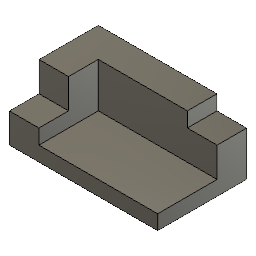
_Practice2.af6316e0-147c-47ba-990e-6d72fd886336 (Autodesk Fusion 360 design; units mm, degrees)
Autodesk Fusion 360 part; units mm, degrees
sketch "Sketch1" plane through (0, 0, 0) normal (0, 0, 1) x (1, 0, 0)
  line L0 (4, 0) -> (0, 0)
  line L1 (0, 0) -> (0, 2.25)
  line L2 (0, 2.25) -> (1.5, 2.25)
  line L3 (1.5, 2.25) -> (1.5, 1.5)
  line L4 (1.5, 1.5) -> (2.75, 1.5)
  line L5 (2.75, 1.5) -> (2.75, 0.75)
  line L6 (2.75, 0.75) -> (4, 0.75)
  line L7 (4, 0.75) -> (4, 0)
  dimension "d1" = 4
  dimension "d4" = 2.25
  dimension "d5" = 1.25
  dimension "d6" = 1.5
  dimension "d7" = 0.75
  dimension "d8" = 0.75
  dimension "d10" = 1.25
  measures "d1" distance of L0.end
  measures "d4" distance of L0.end
sketch "Sketch2" plane through (0, 2.25, 0) normal (0, 1, 0) x (-1, 0, 0)
  line L0 (-1.5, 0) -> (0, 0)
  line L1 (0, 0) -> (0, 1.25)
  line L2 (0, 1.25) -> (-1.5, 1.25)
  line L3 (-1.5, 1.25) -> (-1.5, 0)
  line L4 (-1.5, 0.2963) -> (-0.6318, 0.2963)
  line L5 (-0.6318, 0.2963) -> (-0.6318, 0.976)
  line L6 (-0.6318, 0.976) -> (-3.3284, 0.976)
  line L7 (-3.3284, 0.976) -> (-3.3284, 0.2963)
  line L8 (-3.3284, 0.2963) -> (-1.5, 0.2963)
sketch "Sketch3" plane through (0, 0, 0) normal (0, 0, 1) x (1, 0, 0)
  line L0 (0, 0) -> (100, 0)
  line L1 (100, 0) -> (100, 40)
  line L2 (100, 40) -> (0, 40)
  line L3 (0, 40) -> (0, 0)
  dimension "d15" = 100
  dimension "d16" = 40
extrude "Extrude3" add sketch "Sketch3" along normal blind 60
sketch "Sketch4" plane through (0, 40, 0) normal (0, 1, 0) x (-1, 0, 0)
  line L0 (-100, 0) -> (0, 0)
  line L1 (0, 0) -> (0, 60)
  line L2 (0, 60) -> (-100, 60)
  line L3 (-100, 60) -> (-100, 0)
  line L4 (-20, 60) -> (-20, 20)
  line L5 (-20, 20) -> (-100, 20)
  dimension "d19" = 40
  dimension "d20" = 80
  measures "d19" distance of L0.end
extrude "Extrude4" cut sketch "Sketch4" against normal blind 30 contours L2 L3 L4 L5
sketch "Sketch5" plane through (0, 40, 0) normal (0, 1, 0) x (-1, 0, 0)
  line L0 (-20, 60) -> (-20, 20)
  line L1 (-20, 20) -> (-100, 20)
  line L2 (-100, 20) -> (-100, 0)
  line L3 (-100, 0) -> (0, 0)
  line L4 (0, 0) -> (0, 60)
  line L5 (0, 60) -> (-20, 60)
  line L6 (-20, 40) -> (0, 40)
extrude "Extrude5" cut sketch "Sketch5" against normal blind 20 contours L0 L4 L5 L6
sketch "Sketch6" plane through (0, 40, 0) normal (0, 1, 0) x (-1, 0, 0)
  line L0 (0, 40) -> (-20, 40)
  line L1 (-20, 40) -> (-20, 20)
  line L2 (-20, 20) -> (-100, 20)
  line L3 (-100, 20) -> (-100, 0)
  line L4 (-100, 0) -> (0, 0)
  line L5 (0, 0) -> (0, 40)
  line L6 (-80, 0) -> (-80, 20)
extrude "Extrude6" cut sketch "Sketch6" against normal blind 10 contours L2 L3 L4 L6
